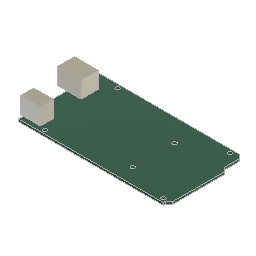
telaioPrincipale v9 (Autodesk Fusion 360 archive; units mm, degrees)
design "arduinoMega"
Autodesk Fusion 360 part; units mm, degrees
sketch "Schizzo1" plane through (0, 0, 0) normal (0, 0, 1) x (1, 0, 0)
  line L0 (25.381, -78.681) -> (25.381, -25.381)
  line L1 (122.0824, -78.681) -> (122.0824, -77.4119)
  line L2 (122.0824, -77.4119) -> (124.6205, -74.8738)
  line L3 (124.6205, -74.8738) -> (124.6205, -40.6095)
  line L4 (25.381, -25.381) -> (119.5443, -25.381)
  line L5 (36.8024, -66.625) -> (23.4774, -66.625)
  line L6 (25.381, -25.381) -> (25.381, -34.8988)
  line L7 (34.8988, -34.8988) -> (19.0357, -34.8988)
  line L8 (25.381, -78.681) -> (122.0824, -78.681)
  line L9 (122.0824, -27.919) -> (122.0824, -38.0714)
  line L10 (122.0824, -27.919) -> (119.5443, -25.381)
  line L11 (124.6205, -40.6095) -> (122.0824, -38.0714)
  line L12 (19.0357, -34.8988) -> (19.0357, -46.3202)
  line L13 (19.0357, -46.3202) -> (34.8988, -46.3202)
  line L14 (34.8988, -46.3202) -> (34.8988, -34.8988)
  line L15 (36.8024, -75.5083) -> (36.8024, -66.625)
  line L16 (23.4774, -66.625) -> (23.4774, -75.5083)
  line L17 (36.8024, -75.5083) -> (23.4774, -75.5083)
  circle A0 centre (40.681, -27.881) radius 1.3
  circle A1 centre (40.681, -76.181) radius 1.3
  circle A2 centre (115.581, -27.881) radius 1.3
  circle A3 centre (119.581, -76.181) radius 1.3
  circle A4 centre (91.481, -68.481) radius 1.3
  circle A5 centre (91.481, -40.581) radius 1.3
  dimension "d30" = 53.3
  dimension "d31" = 94.1633
  dimension "d32" = 15.8631
  dimension "d34" = 9.5179
  dimension "d35" = 6.3452
  dimension "d36" = 25.381
  dimension "d37" = 25.381
  dimension "d40" = 2.5381
  dimension "d41" = 10.1524
  dimension "d43" = 96.7014
  dimension "d44" = 1.269
  dimension "d45" = 2.5381
  dimension "d46" = 34.2643
  dimension "d47" = 2.5381
  dimension "d49" = 2.5381
  dimension "d50" = 2.5381
  dimension "d51" = 2.5381
  dimension "d52" = 11.4214
  dimension "d55" = 13.325
  dimension "d58" = 3.1726
  dimension "d59" = 8.8833
  dimension "d61" = 1.9036
  dimension "d62" = 2.6
  dimension "d63" = 15.3
  dimension "d64" = 2.5
  dimension "d65" = 2.6
  dimension "d66" = 2.5
  dimension "d67" = 15.3
  dimension "d68" = 2.6
  dimension "d69" = 2.5
  dimension "d70" = 74.9
  dimension "d71" = 2.6
  dimension "d72" = 2.5
  dimension "d73" = 78.9
  dimension "d75" = 2.6
  dimension "d76" = 2.6
  dimension "d77" = 50.8
  dimension "d78" = 27.9
  dimension "d79" = 15.2
  constraint vertical L0
  constraint vertical L1
  constraint perpendicular L0 L4
  constraint coincident L5 L16.start
  constraint perpendicular L4 L6
  constraint parallel L4 L8
  constraint parallel L0 L3
  constraint vertical L9
  constraint perpendicular L7 L14
  constraint parallel L12 L14
  constraint perpendicular L13 L14
  constraint parallel L4 L7
  constraint parallel L5 L8
  constraint perpendicular L5 L15
  constraint perpendicular L5 L16
  constraint perpendicular L16 L17
  constraint vertical A4.centre A5.centre
  measures "d30" distance of L0.end L0.start
  measures "d31" distance of L0.end L4.end
  measures "d32" distance of L12.end L13.end
  measures "d34" vertical distance of L0.end L7.end
  measures "d35" horizontal distance of L0.end L7.end
  measures "d36" horizontal distance of origin L0.end
  measures "d37" vertical distance of origin L0.end
  measures "d40" vertical distance of L9.start L4.end
  measures "d41" distance of L9.start L9.end
  measures "d43" distance of L0.start L1.start
  measures "d44" distance of L1.start L1.end
  measures "d45" vertical distance of L2.end L1.end
  measures "d46" distance of L3.end L2.end
  measures "d47" horizontal distance of L1.start L2.end
  measures "d49" horizontal distance of L9.start L4.end
  measures "d50" horizontal distance of L3.end L9.end
  measures "d51" vertical distance of L3.end L9.end
  measures "d52" distance of L12.end L7.end
  measures "d55" distance of L5.start L5.end
  measures "d58" vertical distance of L0.start L15.start
  measures "d59" distance of L5.end L16.end
  measures "d61" horizontal distance of L0.start L16.end
  measures "d62" diameter of A0
  measures "d63" horizontal distance of L0.end A0.centre
  measures "d64" vertical distance of L0.end A0.centre
  measures "d65" diameter of A1
  measures "d66" vertical distance of L0.start A1.centre
  measures "d67" horizontal distance of L0.start A1.centre
  measures "d68" diameter of A2
  measures "d69" vertical distance of L4.end A2.centre
  measures "d70" distance of A0.centre A2.centre
  measures "d71" diameter of A3
  measures "d72" vertical distance of L1.start A3.centre
  measures "d73" distance of A1.centre A3.centre
  measures "d75" diameter of A4
  measures "d76" diameter of A5
  measures "d77" horizontal distance of A0.centre A5.centre
  measures "d78" vertical distance of A4.centre A5.centre
  measures "d79" vertical distance of L4.end A5.centre
extrude "Estrusione1" add sketch "Schizzo1" along normal blind 1.6 contours L0 L7 L13 L14 | L0 L1 L2 L3 L4 L5 L6 L7 L8 L9 L10 L11 L13 L14 L15 L17 | L0 L5 L15 L17 makes body 1
extrude "Estrusione2" add sketch "Schizzo1" along normal blind 10.9 from surface at 1.6 separate body contours L0 L5 L15 L17 | L0 L5 L16 L17 makes body 2
extrude "Estrusione3" add sketch "Schizzo1" along normal blind 10.9 from surface at 1.6 contours L0 L7 L13 L14 | L0 L7 L12 L13 bodies 1
equation "d62 = 1.3 mm * 2"
